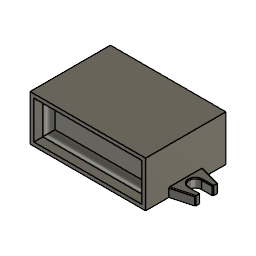
mirror (Autodesk Fusion 360 archive; units mm, degrees)
design "DC-DC Converter"
Autodesk Fusion 360 part; units mm, degrees
sketch "Sketch1" plane through (0, 0, 0) normal (0, 0, 1) x (1, 0, 0)
  line L0 (0, 0) -> (46, 0)
  line L1 (46, 0) -> (46, -32)
  line L2 (46, -32) -> (0, -32)
  line L3 (0, -32) -> (0, 0)
  dimension "d1" = 46
  dimension "d2" = 32
  constraint coincident L0.start L3.end
  constraint horizontal L0
  constraint perpendicular L0 L1
  constraint perpendicular L1 L2
  constraint perpendicular L0 L3
  measures "d1" distance of L0.start L0.end
  measures "d2" distance of L0.end L1.end
extrude "Extrude1" add sketch "Sketch1" along normal blind 18.16
sketch "Sketch2" plane through (0, 0, 0) normal (0, 0, -1) x (1, 0, 0)
  line L0 (46, 32) -> (0, 32)
  line L1 (0, 32) -> (0, 0)
  line L2 (0, 0) -> (46, 0)
  line L3 (46, 0) -> (46, 32)
  line L4 (23, 0) -> (23, 32)
  line L5 (23, 16) -> (-1.31, 16)
  line L6 (23, 16) -> (47.31, 16)
  line L7 (47.31, 16) -> (54.31, 16)
  circle A0 centre (49.81, 16) radius 2.5
  line L8 (-1.31, 16) -> (-8.31, 16)
  circle A1 centre (-3.81, 16) radius 2.5
  line L9 (-8.31, 16) -> (-8.31, 13.5)
  line L10 (-8.31, 16) -> (-8.31, 18.5)
  line L11 (-3.81, 16) -> (-3.81, 18.5)
  line L12 (-3.81, 18.5) -> (-8.31, 18.5)
  line L13 (-3.81, 16) -> (-3.81, 13.5)
  line L14 (-3.81, 13.5) -> (-8.31, 13.5)
  line L15 (49.81, 16) -> (49.81, 18.5)
  line L16 (49.81, 16) -> (49.81, 13.5)
  line L17 (54.31, 16) -> (54.31, 13.5)
  line L18 (49.81, 13.5) -> (54.31, 13.5)
  line L19 (54.31, 16) -> (54.31, 18.5)
  line L20 (49.81, 18.5) -> (54.31, 18.5)
  line L21 (56.31, 16) -> (56.31, 20.5)
  line L22 (47.81, 20.5) -> (56.31, 20.5)
  line L23 (47.81, 16) -> (47.81, 20.5)
  line L24 (47.81, 16) -> (47.81, 11.5)
  line L25 (47.81, 11.5) -> (56.31, 11.5)
  line L26 (56.31, 16) -> (56.31, 11.5)
  line L27 (54.31, 13.5) -> (54.31, 11.5)
  line L28 (-1.81, 16) -> (-1.81, 11.5)
  line L29 (-1.81, 11.5) -> (-10.31, 11.5)
  line L30 (-10.31, 16) -> (-10.31, 11.5)
  line L31 (-10.31, 16) -> (-10.31, 20.5)
  line L32 (-1.81, 20.5) -> (-10.31, 20.5)
  line L33 (-1.81, 16) -> (-1.81, 20.5)
  line L34 (-8.31, 13.5) -> (-8.31, 11.5)
  line L35 (-8.31, 18.5) -> (-8.31, 20.5)
  line L36 (-8.31, 20.5) -> (0, 22.7267)
  line L37 (-8.31, 20.5) -> (0.2931, 20.5) construction
  line L38 (-8.31, 11.5) -> (0, 9.2733)
  line L39 (-8.31, 11.5) -> (0.2931, 11.5) construction
  line L40 (54.31, 11.5) -> (46, 9.2733)
  line L41 (54.31, 11.5) -> (62.9131, 11.5) construction
  line L42 (54.31, 20.5) -> (46, 22.7267)
  line L43 (54.31, 20.5) -> (62.9131, 20.5) construction
  line L44 (54.31, 20.5) -> (54.31, 18.5)
  dimension "d5" = 24.31
  dimension "d6" = 24.31
  dimension "d7" = 7
  dimension "d8" = 5
  dimension "d9" = 7
  dimension "d10" = 5
  dimension "d11" = -2
  dimension "d12" = -2
  dimension "d13" = 15
  dimension "d14" = 15
  dimension "d15" = 165
  dimension "d16" = 165
  constraint midpoint L2 L4.start
  constraint perpendicular L2 L4
  constraint midpoint L4 L5.start
  constraint perpendicular L4 L5
  constraint perpendicular L4 L6
  constraint perpendicular L3 L7
  constraint coincident L6.end A0
  constraint horizontal L8
  constraint coincident L5.end A1
  constraint perpendicular L8 L9
  constraint perpendicular L8 L10
  constraint coincident A1.centre L11.start
  constraint coincident A1 L11.end
  constraint perpendicular L8 L11
  constraint tangent A1 L12
  constraint coincident A1 L13.end
  constraint perpendicular L8 L13
  constraint coincident A0.centre L15.start
  constraint coincident A0 L15.end
  constraint perpendicular L7 L15
  constraint coincident A0 L16.end
  constraint perpendicular L7 L16
  constraint perpendicular L7 L17
  constraint tangent A0 L18
  constraint perpendicular L7 L19
  constraint coincident L25 L27.end
  constraint perpendicular L25 L27
  constraint coincident L29 L34.end
  constraint perpendicular L29 L34
  constraint coincident L32 L35.end
  constraint perpendicular L32 L35
  constraint horizontal L37
  constraint coincident L1 L36.end
  constraint horizontal L39
  constraint coincident L1 L38.end
  constraint horizontal L41
  constraint coincident L3 L40.end
  constraint horizontal L43
  constraint coincident L22 L42.start
  constraint coincident L3 L42.end
  constraint parallel L19 L44
  measures "d5" distance of L5.start L5.end
  measures "d6" distance of L5.start L6.end
  measures "d7" distance of L6.end L7.end
  measures "d8" diameter of A0
  measures "d9" distance of L5.end L8.end
  measures "d10" diameter of A1
  measures "d13" angle of L36 L37
  measures "d14" angle of L38 L39
  measures "d15" angle of L40 L41
  measures "d16" angle of L42 L43
extrude "Extrude2" add sketch "Sketch2" against normal blind 3.5 contours L3 L6 A0 L22 L23 L42 | L3 L6 A0 L24 L25 L40 | A0 L20 L22 L23 L44 | L1 L5 A1 L32 L33 L36 | L1 L5 A1 L28 L29 L38 | A1 L12 L32 L33 L35 | A0 L18 L24 L25 L27 | A1 L14 L28 L29 L34
fillet "Fillet1" radius 0.3 18 edges at (-8.31, -11.5, 1.75) (-8.31, -13.5, 1.75) (-8.31, -18.5, 1.75) (-8.31, -20.5, 1.75) (-6.06, -13.5, 3.5) (-1.31, -16, 3.5) (-6.06, -18.5, 3.5) (-4.155, -10.3867, 3.5) (-4.155, -21.6133, 3.5) (50.155, -10.3867, 3.5) (52.06, -18.5, 3.5) (47.31, -16, 3.5) (52.06, -13.5, 3.5) (54.31, -13.5, 1.75) (54.31, -11.5, 1.75) (54.31, -18.5, 1.75) (54.31, -20.5, 1.75) (50.155, -21.6133, 3.5)
sketch "Sketch3" plane through (0, -32, 0) normal (0, -1, 0) x (1, 0, 0)
  line L0 (0, 0) -> (46, 0)
  line L1 (46, 0) -> (46, 18.16)
  line L2 (46, 18.16) -> (0, 18.16)
  line L3 (0, 18.16) -> (0, 0)
  line L4 (1.5, 1.5) -> (44.5, 1.5)
  line L5 (44.5, 1.5) -> (44.5, 16.66)
  line L6 (44.5, 16.66) -> (1.5, 16.66)
  line L7 (1.5, 16.66) -> (1.5, 1.5)
  dimension "d21" = -1.5
extrude "Extrude3" cut sketch "Sketch3" against normal blind 4.369 contours L4 L5 L6 L7
extrude "Extrude4" cut 1 faces at (15.8333, -27.631, 11.6067) along direction (0, 1, 0) blind 1.648
fillet "Fillet2" radius 2.458 4 edges at (23, -25.983, 1.5) (44.5, -25.983, 9.08) (23, -25.983, 16.66) (1.5, -25.983, 9.08)
equation "d5 = ( 48.62 / 2 ) * 1 mm"
equation "d6 = ( 48.62 / 2 ) * 1 mm"

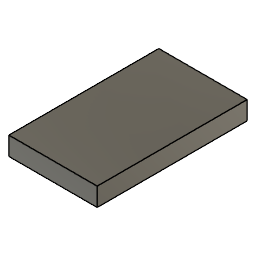
design "TV"
Autodesk Fusion 360 part; units mm, degrees
sketch "Sketch1" plane through (0, 0, 0) normal (0, 0, 1) x (1, 0, 0)
  line L0 (-464.6171, 93.2704) -> (-129.3371, 93.2704)
  line L1 (-129.3371, 93.2704) -> (-129.3371, 691.5253)
  line L2 (-129.3371, 691.5253) -> (-464.6171, 691.5253)
  line L3 (-464.6171, 691.5253) -> (-464.6171, 93.2704)
  line L4 (-464.6171, 691.5253) -> (-129.3371, 93.2704)
  line L5 (-474.1421, 701.0503) -> (-474.1421, 83.7454)
  line L6 (-474.1421, 83.7454) -> (-119.8121, 83.7454)
  line L7 (-119.8121, 83.7454) -> (-119.8121, 701.0503)
  line L8 (-119.8121, 701.0503) -> (-474.1421, 701.0503)
  line L9 (-119.8121, 701.0503) -> (-110.2871, 701.0503)
  line L10 (-110.2871, 701.0503) -> (-110.2871, 59.2786)
  line L11 (-119.8121, 83.7454) -> (-110.2871, 83.7454)
  dimension "d3" = 685.8
  dimension "d11" = 335.28
  dimension "d12" = 9.525
  dimension "d13" = 9.525
  constraint horizontal L0
  constraint vertical L1
  constraint horizontal L2
  constraint vertical L3
  constraint perpendicular L7 L9
  constraint perpendicular L8 L10
  constraint coincident L10 L11.end
  constraint perpendicular L10 L11
  measures "d3" distance of L0.end L2.end
  measures "d11" distance of L0.start L0.end
  measures "d13" distance of L7.end L9.end
extrude "Extrude4" add sketch "Sketch1" along normal blind 76.2 contours L0 L3 L4 | L1 L2 L4 | L5 L6 L7 L8 | L7 L9 L10 L11
sketch "Sketch2" plane through (0, 0, 0) normal (0, 1, 0) x (1, 0, 0)
sketch "Sketch3" plane through (0, 0, 0) normal (0, 1, 0) x (1, 0, 0)
extrude "Extrude1" [rolled back] along distance 76.2 taper angle 0
sketch "Sketch4" plane through (0, 0, 0) normal (0, -1, 0) x (1, 0, 0)
  line L0 (0, 0) -> (434.34, 0)
  line L1 (434.34, 0) -> (434.34, 76.2)
  line L2 (434.34, 76.2) -> (0, 76.2)
  line L3 (0, 76.2) -> (0, 0)
  spline S0 degree 5 poles (434.34, 29.5929) (427.25, 32.8867) (412.7939, 39.2251) (390.2814, 47.9852) (358.5813, 58.1459) (315.9778, 68.1588) (270.1919, 75.2995) (221.0715, 79.4308) (168.7048, 80.6323) (113.3587, 79.1448) (55.3291, 75.2353) (6.9649, 70.3565) (-30.3249, 65.7797) (-55.6292, 62.3275) (-68.3925, 60.501) knots 0 0 0 0 0 0 0.1 0.2 0.3 0.4 0.5 0.6 0.7 0.8 0.9 1 1 1 1 1 1
  point P0 (254, 76.2)
  constraint coincident L1 S0.start
  constraint coincident L2 P0
extrude "Extrude2" [rolled back] along distance -850.7569 taper angle 0
sketch "Sketch5" plane through (0, 0, 0) normal (0, -1, 0) x (1, 0, 0)
  spline S0 degree 5 poles (434.34, 29.5929) (427.25, 32.8867) (412.7939, 39.2251) (390.2814, 47.9852) (358.5813, 58.1459) (321.7709, 66.7973) (291.7271, 71.8631) (269.8442, 74.6015) (257.1058, 75.9003) (254, 76.2) knots 0 0 0 0 0 0 0.1 0.2 0.3 0.4 0.432012 0.432012 0.432012 0.432012 0.432012 0.432012
  line L0 (254, 76.2) -> (0, 76.2)
  line L1 (0, 76.2) -> (0, 0)
  line L2 (0, 0) -> (434.34, 0)
  line L3 (434.34, 0) -> (434.34, 29.5929)
  line L4 (0, 38.1) -> (50.8, 76.2)
  constraint midpoint L1 L4.start
  constraint coincident L0 L4.end
extrude "Extrude3" [rolled back] along distance -910.3614 taper angle 0
